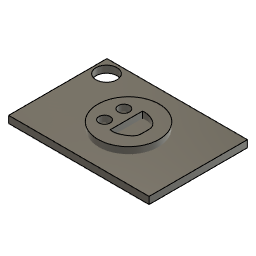
breloc (Autodesk Fusion 360 design; units mm, degrees)
Autodesk Fusion 360 part; units mm, degrees
sketch "Sketch1" plane through (0, 0, 0) normal (0, 1, 0) x (1, 0, 0)
  line L0 (-1.0252, -22.1569) -> (98.9748, -22.1569)
  line L1 (98.9748, -22.1569) -> (98.9748, -92.1569)
  line L2 (98.9748, -92.1569) -> (-1.0252, -92.1569)
  line L3 (-1.0252, -92.1569) -> (-1.0252, -22.1569)
  line L4 (8.9748, -32.1569) -> (88.9748, -32.1569)
  line L5 (88.9748, -32.1569) -> (88.9748, -82.1569)
  line L6 (88.9748, -82.1569) -> (8.9748, -82.1569)
  line L7 (8.9748, -82.1569) -> (8.9748, -32.1569)
  dimension "d1" = 70
  dimension "d2" = 10
  constraint horizontal L0
  constraint vertical L1
  constraint horizontal L2
  constraint vertical L3
  measures "d1" distance of L0.start L2.end
extrude "Extrude1" add sketch "Sketch1" along normal blind 5 contours L0 L1 L2 L3 | L4 L5 L6 L7 makes body 1
move_body "Move1" bodies 1 to x (0, 1, 0) y (-1, 0, 0) z (0, 0, 1) at (63.553, 3.3027, -2.2719)
hole "Hole1" at (63.553, 93.1112, 29.3509) direction (-1, 0, 0) diameter 15 depth 40 tip angle 118 bodies 1
sketch "Sketch2" plane through (0, 0, 0) normal (0, 1, 0) x (1, 0, 0)
  circle A0 centre (135.4066, 179.4915) radius 21.775
extrude "Extrude2" add sketch "Sketch2" along normal blind 5 separate body makes body 2
hole "Hole2" at (145.1913, 5, -186.8161) direction (0, -1, 0) diameter 8 depth 5 tip angle 118 bodies 2
hole "Hole3" at (145.0712, 5, -173.1534) direction (0, -1, 0) diameter 8 depth 5 tip angle 118 bodies 2
sketch "Sketch3" plane through (0, 0, 0) normal (0, 1, 0) x (1, 0, 0)
hole "Hole4" at (130.0467, 5, -180.1312) direction (0, -1, 0) diameter 12 depth 5 tip angle 118 bodies 2
sketch "Sketch4" plane through (0, 0, 0) normal (0, 1, 0) x (1, 0, 0)
  line L0 (137, 191) -> (137, 168.502)
  spline S0 degree 5 poles (137, 191) (136.82, 191.0301) (136.4621, 191.0834) (135.9322, 191.1427) (135.2391, 191.1805) (134.3937, 191.1583) (133.5638, 191.0656) (132.7388, 190.9004) (131.8998, 190.6598) (131.0244, 190.3399) (130.0944, 189.9374) (129.1035, 189.4498) (128.0637, 188.8762) (127.0145, 188.2185) (126.0137, 187.481) (125.1236, 186.6697) (124.3997, 185.7927) (123.8789, 184.859) (123.5654, 183.8788) (123.4229, 182.8629) (123.3935, 181.8219) (123.4134, 180.7663) (123.4304, 179.705) (123.42, 178.6457) (123.4023, 177.5935) (123.4246, 176.5529) (123.5472, 175.5283) (123.8269, 174.5257) (124.3025, 173.5536) (124.9781, 172.6245) (125.8297, 171.7531) (126.8154, 170.9545) (127.8841, 170.2425) (128.9839, 169.6274) (130.072, 169.1144) (131.1222, 168.7018) (132.1209, 168.3834) (133.0636, 168.15) (133.9517, 167.992) (134.7886, 167.9007) (135.5769, 167.8708) (136.1696, 167.8937) (136.593, 167.9368) (136.8659, 167.977) (137, 168) knots 0 0 0 0 0 0 0.025 0.05 0.075 0.1 0.125 0.15 0.175 0.2 0.225 0.25 0.275 0.3 0.325 0.35 0.375 0.4 0.425 0.45 0.475 0.5 0.525 0.55 0.575 0.6 0.625 0.65 0.675 0.7 0.725 0.75 0.775 0.8 0.825 0.85 0.875 0.9 0.925 0.95 0.975 1 1 1 1 1 1
  line L1 (137, 168.502) -> (137, 168)
  point P0 (133.2868, 191)
  point P1 (128.9287, 189.3422)
  point P2 (124, 185)
  point P3 (123.4238, 179.751)
  point P4 (123.9153, 174.4329)
  point P5 (128.8632, 169.7144)
  point P6 (134, 168)
  constraint vertical L0
  constraint parallel L0 L1
extrude "Extrude3" cut sketch "Sketch4" along normal blind 5 bodies 2
move_body "Move2" bodies 2 to x (1, 0, 0) y (0, 1, 0) z (0, 0, 1) at (-60, 0, 80)
move_body "Move3" bodies 2 to x (1, 0, 0) y (0, 1, 0) z (0, 0, 1) at (-50, 0, 80)
move_body "Move4" bodies 1 to x (0, 1, 0) y (-1, 0, 0) z (0, 0, 1) at (156.6642, -52.9418, 0)
move_body "Move5" bodies 2 to x (-1, 0, 0) y (0, 1, 0) z (0, 0, -1) at (130.8131, 10, 36.017)
move_body "Move6" bodies 1 2 to x (1, 0, 0) y (0, 1, 0) z (0, 0, 1) at (0, -5, 0)
